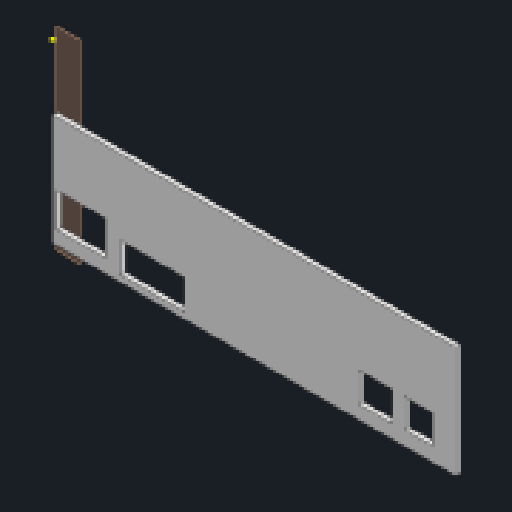
# Autodesk Inventor part: ceil_front
Saved by Autodesk Inventor 2023 (Build 270158000, 158)
## iProperties
Created: 2024-04-28
Part Number: ceil_front
Material: Generic
Document SubType Name: Modeling
Designer: szymo
Density: 1 g/cm^3
Appearance: Default
Author: szymo
Autodesk Inventor part; units mm, degrees
ref_plane "YZ Plane" through (0, 0, 0) normal (1, 0, 0) x (0, 1, 0)
ref_plane "XZ Plane" through (0, 0, 0) normal (0, 1, 0) x (-1, 0, 0)
ref_plane "XY Plane" through (0, 0, 0) normal (0, 0, 1) x (1, 0, 0)
ref_plane "Work Plane1" through (0, 0, 0) normal (0, 0, 1) x (1, 0, 0)
sketch "Sketch1" plane through (0, 0, 0) normal (0, 0, 1) x (1, 0, 0)
  circle A0 centre (118.7, -21.5445) radius 2.5 projected
  circle A1 centre (113.95, -8.8843) radius 2.5 projected
  circle A2 centre (64.05, -19.8657) radius 2.5 projected
  circle A3 centre (59.3, -7.2055) radius 2.5 projected
  circle A4 centre (64.05, -8.8843) radius 2.5 projected
  circle A5 centre (59.3, -21.5445) radius 2.5 projected
  circle A6 centre (118.7, -7.2055) radius 2.5 projected
  circle A7 centre (113.95, -19.8657) radius 2.5 projected
  line L0 (84.5, 12.4325) -> (84.5, -11.5675) projected
  line L1 (84.5, -11.5675) -> (72.5, -11.5675) projected
  line L2 (72.5, -11.5675) -> (72.5, 4.5875) projected
  circle A8 centre (69.5, 4.5875) radius 3 projected
  line L3 (72.5, 4.5875) -> (72.5, 12.4325) projected
  line L4 (72.5, 12.4325) -> (84.5, 12.4325) projected
  arc A9 (105.5, 4.2836) -> (105.5, 4.8914) centre (108.4846, 4.5875) ccw projected
  line L5 (105.5, 4.2836) -> (105.5, -11.5675) projected
  line L6 (105.5, -11.5675) -> (93.5, -11.5675) projected
  line L7 (93.5, -11.5675) -> (93.5, 12.4325) projected
  line L8 (93.5, 12.4325) -> (105.5, 12.4325) projected
  line L9 (105.5, 12.4325) -> (105.5, 4.8914) projected
  circle A10 centre (108.4462, 27.5) radius 3 projected
  circle A11 centre (69.5, 27.5) radius 3 projected
  circle A12 centre (89, 0.9661) radius 3 projected
  circle A13 centre (89, 29.5) radius 3 projected
  arc A14 (175, 0) -> (178, -3) centre (175, -3) ccw projected
  line L10 (175, 0) -> (112.5, 0) projected
  line L11 (112.5, 0) -> (112.5, 55) projected
  line L12 (112.5, 55) -> (65.5, 55) projected
  line L13 (65.5, 55) -> (65.5, 0) projected
  line L14 (65.5, 0) -> (3, 0) projected
  arc A15 (0, -3) -> (3, 0) centre (3, -3) ccw projected
  line L15 (0, -3) -> (0, -25.75) projected
  arc A16 (3, -28.75) -> (0, -25.75) centre (3, -25.75) ccw projected
  line L16 (3, -28.75) -> (175, -28.75) projected
  arc A17 (178, -25.75) -> (175, -28.75) centre (175, -25.75) ccw projected
  line L17 (178, -25.75) -> (178, -3) projected
  circle A18 centre (3, -25.75) radius 2.3 projected
  circle A19 centre (3, -3) radius 2.3 projected
  circle A20 centre (3, -74.8889) radius 2.3 projected
  line L18 (0, 0) -> (6, 0) projected
  line L19 (0, -77.8889) -> (0, 0) projected
  line L20 (0, -77.8889) -> (6, -77.8889) projected
  line L21 (6, -71.8889) -> (6, -77.8889) projected
  line L22 (6, -71.8889) -> (1.6, -71.8889) projected
  line L23 (1.6, -71.8889) -> (1.6, -56.7889) projected
  line L24 (1.6, -56.7889) -> (9.6, -56.7889) projected
  line L25 (9.6, -44.7889) -> (9.6, -56.7889) projected
  line L26 (3, -44.7889) -> (9.6, -44.7889) projected
  line L27 (3, -28.75) -> (3, -44.7889) projected
  line L28 (3, -28.75) -> (6, -28.75) projected
  line L29 (6, -28.75) -> (6, -22.75) projected
  line L30 (6, -22.75) -> (3, -22.75) projected
  line L31 (3, -6) -> (3, -22.75) projected
  line L32 (3, -6) -> (6, -6) projected
  line L33 (6, -6) -> (6, 0) projected
  circle A21 centre (5.6, -52.7889) radius 2.6 projected
  circle A22 centre (175, -3) radius 2.3 projected
  circle A23 centre (175, -25.75) radius 2.3 projected
  line L34 (175, -28.75) -> (175, -41.8889) projected
  line L35 (168.4, -41.8889) -> (175, -41.8889) projected
  line L36 (168.4, -53.8889) -> (168.4, -41.8889) projected
  line L37 (175, -53.8889) -> (168.4, -53.8889) projected
  line L38 (175, -53.8889) -> (175, -71.8889) projected
  line L39 (175, -71.8889) -> (172, -71.8889) projected
  line L40 (172, -71.8889) -> (172, -77.8889) projected
  line L41 (178, -77.8889) -> (172, -77.8889) projected
  line L42 (178, -77.8889) -> (178, 0) projected
  line L43 (178, 0) -> (172, 0) projected
  line L44 (172, 0) -> (172, -6) projected
  line L45 (172, -6) -> (175, -6) projected
  line L46 (175, -6) -> (175, -22.75) projected
  line L47 (175, -22.75) -> (172, -22.75) projected
  line L48 (172, -22.75) -> (172, -28.75) projected
  line L49 (172, -28.75) -> (175, -28.75) projected
  circle A24 centre (175, -74.8889) radius 2.3 projected
  circle A25 centre (172.4, -49.8889) radius 2.6 projected
  line L50 (156.2, -70.4889) -> (156.2, -59.9889) projected
  line L51 (166.7, -59.9889) -> (156.2, -59.9889) projected
  line L52 (166.7, -59.9889) -> (166.7, -70.4889) projected
  line L53 (156.2, -70.4889) -> (166.7, -70.4889) projected
  line L54 (149, -59.8889) -> (149, -70.8889) projected
  line L55 (149, -70.8889) -> (136.35, -70.8889) projected
  line L56 (136.35, -70.8889) -> (136.35, -59.8889) projected
  line L57 (136.35, -59.8889) -> (149, -59.8889) projected
  line L58 (135, -53.8889) -> (135, -71.8889) projected
  line L59 (135, -71.8889) -> (175, -71.8889) projected
  line L60 (175, -71.8889) -> (175, -53.8889) projected
  line L61 (175, -53.8889) -> (135, -53.8889) projected
  circle A26 centre (137.85, -56.7389) radius 1.5 projected
  circle A27 centre (172.15, -56.7389) radius 1.5 projected
  line L62 (31.25, -62.8889) -> (31.25, -73.8889) projected
  line L63 (31.25, -73.8889) -> (57.25, -73.8889) projected
  line L64 (57.25, -73.8889) -> (57.25, -62.8889) projected
  line L65 (57.25, -62.8889) -> (31.25, -62.8889) projected
  line L66 (9.6, -56.7889) -> (23.3, -56.7889) projected
  line L67 (23.3, -56.7889) -> (23.3, -59.8889) projected
  line L68 (23.3, -59.8889) -> (23.3, -65.1889) projected
  line L69 (3, -71.8889) -> (23.3, -71.8889) projected
  line L70 (23.3, -61.8889) -> (23.3, -74.8889) projected
  line L71 (30.25, -61.8889) -> (30.25, -74.8889)
  line L72 (30.25, -74.8889) -> (58.25, -74.8889)
  line L73 (58.25, -74.8889) -> (58.25, -61.8889)
  line L74 (58.25, -61.8889) -> (30.25, -61.8889)
  line L75 (150, -58.8889) -> (150, -71.8889)
  line L76 (150, -71.8889) -> (135.35, -71.8889)
  line L77 (135.35, -71.8889) -> (135.35, -58.8889)
  line L78 (135.35, -58.8889) -> (150, -58.8889)
  line L79 (155.2, -58.9889) -> (155.2, -71.4889)
  line L80 (155.2, -71.4889) -> (167.7, -71.4889)
  line L81 (167.7, -71.4889) -> (167.7, -58.9889)
  line L82 (167.7, -58.9889) -> (155.2, -58.9889)
  line L83 (0, -28.75) -> (178, -28.75)
  line L84 (178, -28.75) -> (178, -77.8889)
  line L85 (178, -77.8889) -> (0, -77.8889)
  line L86 (0, -77.8889) -> (0, -28.75)
  point P0 (3, -28.75)
  point P1 (175, -28.75)
  point P2 (135.35, -71.8889)
  dimension "d0" = 1
  dimension "d1" = 1
  dimension "d2" = 1
  constraints: 32 end point, 2 parallel, 1 horizontal, 1 horizontal alignment, 1 perpendicular, 1 point on line, 9 other
  measures "d0" distance between parallel lines of L65 L74
  measures "d1" distance between parallel lines of L57 L78
  measures "d2" distance between parallel lines of L51 L82
extrude "Extrusion1" add sketch "Sketch1" along normal blind 2 contours L42 L41 L40 L39 L38 L37 L36 L35 L34 L83 | L34 L35 L36 L61 L58 L59 L40 L85 L21 L69 L70 L68 L67 L66 L25 L26 L27 L16 | L27 L26 L25 L24 L23 L22 L21 L20 L19 L83 | L59 L75 L78 L77 L58 L61 L37 L38 L39 | A20 | A21 | A24 | A25 | A26 | A27
sketch "Sketch2" plane through (0, 0, 2) normal (0, 0, 1) x (1, 0, 0)
  circle A0 centre (3, -25.75) radius 2.3 projected
  circle A1 centre (3, -3) radius 2.3 projected
  circle A2 centre (3, -74.8889) radius 2.3 projected
  line L0 (0, 0) -> (6, 0) projected
  line L1 (0, -77.8889) -> (0, 0) projected
  line L2 (0, -77.8889) -> (6, -77.8889) projected
  line L3 (6, -71.8889) -> (6, -77.8889) projected
  line L4 (6, -71.8889) -> (1.6, -71.8889) projected
  line L5 (1.6, -71.8889) -> (1.6, -56.7889) projected
  line L6 (1.6, -56.7889) -> (9.6, -56.7889) projected
  line L7 (9.6, -44.7889) -> (9.6, -56.7889) projected
  line L8 (3, -44.7889) -> (9.6, -44.7889) projected
  line L9 (3, -28.75) -> (3, -44.7889) projected
  line L10 (3, -28.75) -> (6, -28.75) projected
  line L11 (6, -28.75) -> (6, -22.75) projected
  line L12 (6, -22.75) -> (3, -22.75) projected
  line L13 (3, -6) -> (3, -22.75) projected
  line L14 (3, -6) -> (6, -6) projected
  line L15 (6, -6) -> (6, 0) projected
  circle A3 centre (5.6, -52.7889) radius 2.6 projected
  circle A4 centre (172.4, -49.8889) radius 2.6 projected
  circle A5 centre (175, -3) radius 2.3 projected
  circle A6 centre (175, -25.75) radius 2.3 projected
  line L16 (175, -28.75) -> (175, -41.8889) projected
  line L17 (168.4, -41.8889) -> (175, -41.8889) projected
  line L18 (168.4, -53.8889) -> (168.4, -41.8889) projected
  line L19 (175, -53.8889) -> (168.4, -53.8889) projected
  line L20 (175, -53.8889) -> (175, -71.8889) projected
  line L21 (175, -71.8889) -> (172, -71.8889) projected
  line L22 (172, -71.8889) -> (172, -77.8889) projected
  line L23 (178, -77.8889) -> (172, -77.8889) projected
  line L24 (178, -77.8889) -> (178, 0) projected
  line L25 (178, 0) -> (172, 0) projected
  line L26 (172, 0) -> (172, -6) projected
  line L27 (172, -6) -> (175, -6) projected
  line L28 (175, -6) -> (175, -22.75) projected
  line L29 (175, -22.75) -> (172, -22.75) projected
  line L30 (172, -22.75) -> (172, -28.75) projected
  line L31 (172, -28.75) -> (175, -28.75) projected
  circle A7 centre (175, -74.8889) radius 2.3 projected
  circle A8 centre (172.4, -49.8889) radius 2.6 projected
  constraints: 4 coincident
hole "Hole1" at (5.6, -52.7889, 2) at (3, -74.8889, 2) at (175, -74.8889, 2) at (172.4, -49.8889, 2) direction (0, 0, -1) diameter 3.6 end through all countersink diameter 6 countersink angle 90 clearance for "Countersunk Flat Head Screw ISO 2009/7046" size "M3" standard "ISO"
body "Solid1"
